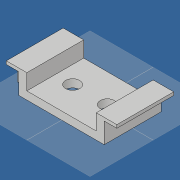
# Autodesk Inventor part: Hutschiene
Saved by Autodesk Inventor 2019 (Build 230136000, 136)
## iProperties
Created: 2020-08-30
Part Number: Hutschiene
Material: Generisch
Document SubType Name: Modeling
Designer: Stefan
Mass: 2.01548 g
Surface Area: 19.7007 cm^2
Volume: 2.01548 cm^3
Density: 1 g/cm^3
Appearance: Vorgabe
Author: Stefan
Autodesk Inventor part; units mm, degrees
ref_plane "YZ Plane" through (0, 0, 0) normal (1, 0, 0) x (0, 1, 0)
ref_plane "XZ Plane" through (0, 0, 0) normal (0, 1, 0) x (-1, 0, 0)
ref_plane "XY Plane" through (0, 0, 0) normal (0, 0, 1) x (1, 0, 0)
sketch "Skizze1" plane through (0, 0, 0) normal (0, 0, 1) x (1, 0, 0)
  line L0 (-17.5, 7.5) -> (-17.5, 6.5)
  line L1 (-17.5, 6.5) -> (-13.5, 6.5)
  line L2 (-13.5, 6.5) -> (-13.5, 0)
  line L3 (-13.5, 0) -> (13.5, 0)
  line L4 (13.5, 0) -> (13.5, 6.5)
  line L5 (13.5, 6.5) -> (17.5, 6.5)
  line L6 (17.5, 6.5) -> (17.5, 7.5)
  line L7 (17.5, 7.5) -> (11, 7.5)
  line L8 (-11, 7.5) -> (-17.5, 7.5)
  line L9 (0, -1.5) -> (0, 9) construction
  line L10 (-11, 2.5) -> (11, 2.5)
  line L11 (-11, 7.5) -> (-11, 2.5)
  line L12 (11, 2.5) -> (11, 7.5)
  line L13 (-13.5, 0) -> (-17.5, 0)
  line L14 (-17.5, 0) -> (-17.5, 6.5)
  line L15 (-17.5, 6.5) -> (-13.5, 6.5)
  line L16 (-13.5, 6.5) -> (-13.5, 0)
  point P0 (0, 0)
  point P1 (0, 2.5)
  dimension "d0" = 1
  dimension "d1" = 35
  dimension "d2" = 27
  dimension "d3" = 7.5
  dimension "d6" = 4
  dimension "d7" = 2.5
  dimension "d8" = 2.5
  constraints: 32 end point, 7 perpendicular, 4 point on line, 3 vertical, 2 horizontal, 2 midpoint, 2 parallel, 2 other
  measures "d0" distance between parallel lines of L1 L8
  measures "d1" distance between parallel lines of L6 L0
  measures "d2" distance between parallel lines of L4 L2
  measures "d3" distance between parallel lines of L3 L8
  measures "d6" distance between parallel lines of L2 L0
  measures "d7" distance between parallel lines of L11 L2
  measures "d8" distance between parallel lines of L3 L10
extrude "Extrusion1" add sketch "Skizze1" along normal mid plane 18 contours L8 L11 L10 L12 L7 L6 L5 L4 L3 L2 L1 L0
extrude "Extrusion2" add sketch "Skizze1" along normal mid plane 11 contours L1 L2 L13 L14
sketch "Skizze2" plane through (-11, 2.5, 9) normal (0, 1, 0) x (1, 0, 0)
  line L0 (0, 18) -> (0, 0) projected
  line L1 (22, 0) -> (0, 0) projected
  line L2 (22, 18) -> (22, 0) projected
  line L3 (0, 18) -> (22, 18) projected
  line L4 (0, 9) -> (22, 9) construction
  line L5 (11, 0) -> (11, 18) construction
  point P0 (11, 9)
  point P1 (5.5, 9)
  point P2 (16.5, 9)
  dimension "d13" = 11
  dimension "d14" = 22
  constraints: 4 end point, 4 midpoint, 2 point on line, 1 symmetric about line
  measures "d13" distance of point (16.5, 9) point (5.5, 9)
  measures "d14" distance between parallel lines of L2 L0
hole "Bohrung1" at (-5.5, 2.5, 0) at (5.5, 2.5, 0) direction (0, -1, 0) diameter 4.5 end through all clearance for "Flachkopfsenkschraube DIN EN ISO 2009" size "M4" standard "DIN"
